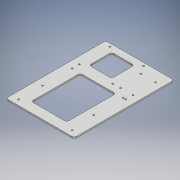
# Autodesk Inventor part: Платформа для контроллера PERCo
Saved by Autodesk Inventor 2018 (Build 220112000, 112)
## iProperties
Created: 2019-04-04
Part Number: Платформа для контроллера PERCo
Material: Типовые
Document SubType Name: Modeling
Designer: KV33_HP1
Density: 1 g/cm^3
Appearance: По умолчанию
Author: KV33_HP1
Autodesk Inventor part; units mm, degrees
ref_plane "YZ Plane" through (0, 0, 0) normal (1, 0, 0) x (0, 1, 0)
ref_plane "XZ Plane" through (0, 0, 0) normal (0, 1, 0) x (-1, 0, 0)
ref_plane "XY Plane" through (0, 0, 0) normal (0, 0, 1) x (1, 0, 0)
sketch "Эскиз1" plane through (0, 0, 0) normal (0, 0, 1) x (1, 0, 0)
  circle A0 centre (5, 5) radius 1.6
  circle A1 centre (115, 5) radius 1.6
  circle A2 centre (115, 115) radius 1.6
  circle A3 centre (5, 115) radius 1.6
  circle A4 centre (115, 130) radius 1.6
  circle A5 centre (89.5, 130) radius 1.6
  circle A6 centre (115, 176) radius 1.6
  circle A7 centre (85, 176) radius 1.6
  line L0 (5, 126) -> (1, 126)
  circle A8 centre (5, 192.5) radius 1.6
  circle A9 centre (74, 192.5) radius 1.6
  circle A10 centre (74, 129.5) radius 1.6
  circle A11 centre (5, 129.5) radius 1.6
  circle A12 centre (5, 54) radius 1.6
  circle A13 centre (110, 54) radius 1.6
  circle A14 centre (110, 115) radius 1.6
  line L1 (-10, -1) -> (-10, 194)
  line L2 (-5, 199) -> (125, 199)
  line L3 (130, 194) -> (130, -1)
  line L4 (-5, -6) -> (125, -6)
  arc A15 (-5, 199) -> (-10, 194) centre (-5, 194) ccw
  arc A16 (130, 194) -> (125, 199) centre (125, 194) ccw
  arc A17 (125, -6) -> (130, -1) centre (125, -1) ccw
  arc A18 (-10, -1) -> (-5, -6) centre (-5, -1) ccw
  line L5 (26.34, 115) -> (89.5732, 115)
  line L6 (94.5732, 110) -> (94.5732, 19.2374)
  line L7 (89.5732, 14.2374) -> (26.34, 14.2374)
  line L8 (21.34, 19.2374) -> (21.34, 110)
  line L9 (58.0791, 137.9369) -> (21.4072, 137.9369)
  line L10 (16.4072, 142.9369) -> (16.4072, 179.6089)
  line L11 (21.4072, 184.6089) -> (58.0791, 184.6089)
  line L12 (63.0791, 179.6089) -> (63.0791, 142.9369)
  arc A19 (21.4072, 184.6089) -> (16.4072, 179.6089) centre (21.4072, 179.6089) ccw
  arc A20 (63.0791, 179.6089) -> (58.0791, 184.6089) centre (58.0791, 179.6089) ccw
  arc A21 (58.0791, 137.9369) -> (63.0791, 142.9369) centre (58.0791, 142.9369) ccw
  arc A22 (16.4072, 142.9369) -> (21.4072, 137.9369) centre (21.4072, 142.9369) ccw
  arc A23 (26.34, 115) -> (21.34, 110) centre (26.34, 110) ccw
  arc A24 (21.34, 19.2374) -> (26.34, 14.2374) centre (26.34, 19.2374) ccw
  arc A25 (89.5732, 14.2374) -> (94.5732, 19.2374) centre (89.5732, 19.2374) ccw
  arc A26 (94.5732, 110) -> (89.5732, 115) centre (89.5732, 110) ccw
  point P0 (0, 0)
  point P1 (-10, -6)
  point P2 (-10, 199)
  dimension "d6" = 3.2
  dimension "d7" = 3.2
  dimension "d8" = 3.2
  dimension "d9" = 3.2
  dimension "d11" = 3.2
  dimension "d13" = 3.2
  dimension "d15" = 3.2
  dimension "d17" = 3.2
  dimension "d18" = 11
  dimension "d19" = 4
  dimension "d25" = 3.2
  dimension "d26" = 3.2
  dimension "d30" = 3.2
  dimension "d31" = 3.2
  dimension "d32" = 3.2
  dimension "d35" = 205
  dimension "d37" = 5
  dimension "d38" = 5
  constraints: 27 centre point, 26 end point, 24 point on circle, 24 tangent, 10 equal radius, 5 horizontal, 4 parallel, 4 point on line, 3 perpendicular
  measures "d6" diameter of A0
  measures "d7" diameter of A1
  measures "d8" diameter of A2
  measures "d9" diameter of A3
  measures "d11" diameter of A4
  measures "d13" diameter of A5
  measures "d15" diameter of A6
  measures "d17" diameter of A7
  measures "d18" distance of A3.centre L0.start
  measures "d19" distance of L0.start L0.end
  measures "d25" diameter of A8
  measures "d26" diameter of A10
  measures "d30" diameter of A12
  measures "d31" diameter of A13
  measures "d32" diameter of A14
  measures "d35" distance of point (-10, -6) point (-10, 199)
  measures "d37" radius of A15
  measures "d38" radius of A19
extrude "Выдавливание1" add sketch "Эскиз1" along normal blind 3
